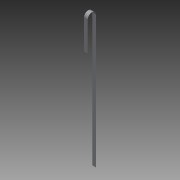
# Autodesk Inventor part: guide
Saved by Autodesk Inventor 2013 (Build 170138000, 138)
## iProperties
Created: 2013-01-17
Part Number: guide
Material: Generic
Document SubType Name: Modeling
Designer: istvan.burbank
Density: 1 g/cm^3
Author: istvan.burbank
Autodesk Inventor part; units mm, degrees
ref_plane "YZ Plane" through (0, 0, 0) normal (1, 0, 0) x (0, 1, 0)
ref_plane "XZ Plane" through (0, 0, 0) normal (0, 1, 0) x (-1, 0, 0)
ref_plane "XY Plane" through (0, 0, 0) normal (0, 0, 1) x (1, 0, 0)
sketch "Sketch1" plane through (0, 0, 0) normal (1, 0, 0) x (0, 1, 0)
  line L0 (708.8975, 55.88) -> (914.4, 55.88)
  arc A0 (914.4, 0) -> (914.4, 55.88) centre (914.4, 27.94) ccw
  line L1 (914.4, 0) -> (0, 0)
  line L2 (708.8975, 56.134) -> (914.4, 56.134)
  arc A1 (914.4, -0.254) -> (914.4, 56.134) centre (914.4, 27.94) ccw
  line L3 (914.4, -0.254) -> (0, -0.254)
  line L4 (708.8975, 55.88) -> (708.8975, 56.134)
  line L5 (0, -0.254) -> (0, 0)
  dimension "d6" = 27.94
  dimension "d7" = 914.4
  dimension "d12" = 0.254
  constraints: 12 end point, 4 point on circle, 3 parallel, 2 centre point, 1 coincident, 1 horizontal, 1 perpendicular, 1 tangent, 1 vertical alignment, 2 other
  measures "d6" radius of A0
  measures "d7" horizontal distance of A0.centre point (0, 0)
  measures "d12" distance of L3.end L1.end
extrude "Extrusion2" add sketch "Sketch1" against normal blind 25.4
body "Solid3"
